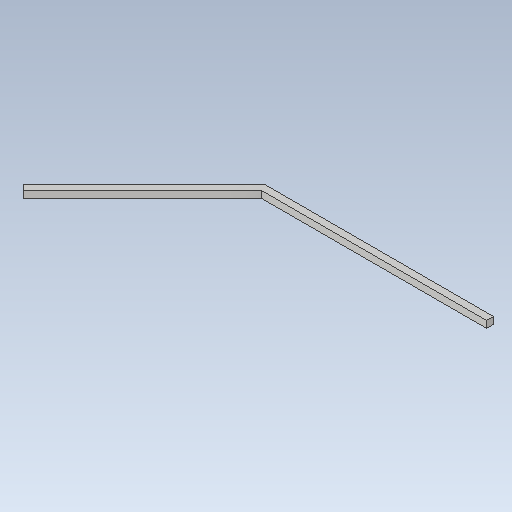
# Autodesk Inventor part: A_LeftWall1(plan)_5
Saved by Autodesk Inventor 2020 (Build 240168000, 168)
## iProperties
Created: 2020-12-21
Part Number: A_LeftWall1(plan)_5
Material: Generic
Document SubType Name: Modeling
Designer: Dell
Density: 1 g/cm^3
Appearance: Default
Author: Dell
Autodesk Inventor part; units mm, degrees
ref_plane "YZ Plane" through (0, 0, 0) normal (1, 0, 0) x (0, 1, 0)
ref_plane "XZ Plane" through (0, 0, 0) normal (0, 1, 0) x (-1, 0, 0)
ref_plane "XY Plane" through (0, 0, 0) normal (0, 0, 1) x (1, 0, 0)
sketch "Sketch1" plane through (0, 0, 0) normal (0, 1, 0) x (-1, 0, 0)
  line L0 (0, 0) -> (200, 0)
  line L1 (200, 0) -> (306.066, 106.066)
  line L2 (306.066, 106.066) -> (301.8234, 110.3087)
  line L3 (301.8234, 110.3087) -> (197.5147, 6)
  line L4 (0, 0) -> (0, 6)
  line L5 (0, 6) -> (197.5147, 6)
  dimension "d0" = 200
  dimension "d2" = 135
  dimension "d3" = 6
  dimension "d4" = 90
  dimension "d6" = 6
  dimension "d10" = 197.5147
  dimension "d11" = 150
  constraints: 12 end point, 1 horizontal, 1 perpendicular, 1 vertical
  measures "d0" distance of L0.start L0.end
  measures "d2" angle of L1 L0
  measures "d3" distance of L1.end L2.end
  measures "d4" angle of L3 L2
  measures "d6" distance of L0.start L4.end
  measures "d10" distance of L4.end L3.end
  measures "d11" distance of L0.end L1.end
extrude "Extrusion1" add sketch "Sketch1" along normal blind 6
body "Solid1"
